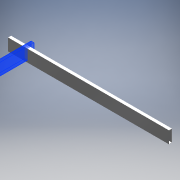
# Autodesk Inventor part: Bumper Plate
Saved by Autodesk Inventor 2019.4 (Build 234330000, 330)
## iProperties
Created: 2019-12-11
Part Number: Bumper Plate
Material: Aluminum 6061
Document SubType Name: Modeling
Designer: Mark
Mass: 315.36 g
Surface Area: 2338.92 cm^2
Volume: 116.8 cm^3
Density: 2.7 g/cm^3
Appearance: Aluminum - Flat
Author: Mark
Autodesk Inventor part; units mm, degrees
ref_plane "YZ Plane" through (0, 0, 0) normal (1, 0, 0) x (0, 1, 0)
ref_plane "XZ Plane" through (0, 0, 0) normal (0, 1, 0) x (-1, 0, 0)
ref_plane "XY Plane" through (0, 0, 0) normal (0, 0, 1) x (1, 0, 0)
sketch "Sketch1" plane through (0, 0, 0) normal (1, 0, 0) x (0, 1, 0)
  line L0 (-30, 7.5) -> (30, 7.5)
  line L1 (30, 7.5) -> (30, -7.5)
  line L2 (30, -7.5) -> (-30, -7.5)
  line L3 (-30, -7.5) -> (-30, 7.5)
  line L4 (-30, 7.5) -> (30, -7.5) construction
  line L5 (30, 7.5) -> (-30, -7.5) construction
  line L6 (-29, 6.5) -> (29, 6.5)
  line L7 (29, 6.5) -> (29, -6.5)
  line L8 (29, -6.5) -> (-29, -6.5)
  line L9 (-29, -6.5) -> (-29, 6.5)
  line L10 (-29, 6.5) -> (29, -6.5) construction
  line L11 (29, 6.5) -> (-29, -6.5) construction
  point P0 (0, 0)
  dimension "d0" = 60
  dimension "d1" = 15
  dimension "d2" = 58
  dimension "d3" = 13
  constraints: 24 end point, 4 midpoint, 4 parallel, 2 horizontal, 2 perpendicular
  measures "d0" distance of L1.end L2.end
  measures "d1" distance of L0.end L1.end
  measures "d2" distance of L7.end L8.end
  measures "d3" distance of L6.end L7.end
extrude "Extrusion1" add sketch "Sketch1" along normal blind 800
sketch "Sketch2" plane through (0, 30, 7.5) normal (0, 1, 0) x (1, 0, 0)
  circle A0 centre (20, 7.5) radius 2.75
  circle A1 centre (780, 7.5) radius 2.75
  circle A2 centre (760, 7.5) radius 2.75
  circle A3 centre (40, 7.5) radius 2.75
  line L0 (0, 0) -> (0, 15) projected
  line L1 (0, 0) -> (800, 0) projected
  line L2 (800, 15) -> (800, 0) projected
  point P0 (0, 7.5)
  dimension "d6" = 5.5
  dimension "d7" = 5.5
  dimension "d8" = 5.5
  dimension "d9" = 5.5
  dimension "d10" = 20
  dimension "d11" = 20
  dimension "d12" = 7.5
  dimension "d13" = 7.5
  dimension "d14" = 7.5
  dimension "d15" = 7.5
  dimension "d16" = 20
  dimension "d17" = 20
  constraints: 4 centre point
  measures "d6" diameter of A0
  measures "d7" diameter of A1
  measures "d8" diameter of A2
  measures "d9" diameter of A3
  measures "d10" distance from line of L0 A0.centre
  measures "d11" distance of A3.centre A0.centre
  measures "d12" distance from line of L1 A0.centre
  measures "d13" distance from line of L1 A3.centre
  measures "d14" distance from line of A2.centre L1
  measures "d15" distance from line of L1 A1.centre
  measures "d16" distance of A2.centre A1.centre
  measures "d17" distance from line of L2 A1.centre
extrude "Extrusion2" cut sketch "Sketch2" against normal blind 800
body "Solid1"
